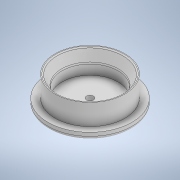
# Autodesk Inventor part: tale
Saved by Autodesk Inventor 2022 (Build 260153000, 153)
## iProperties
Created: 2023-01-18
Part Number: tale
Material: Generic
Document SubType Name: Modeling
Designer: CLCK
Density: 1 g/cm^3
Appearance: Default
Author: CLCK
Autodesk Inventor part; units mm, degrees
ref_plane "YZ Plane" through (0, 0, 0) normal (1, 0, 0) x (0, 1, 0)
ref_plane "XZ Plane" through (0, 0, 0) normal (0, 1, 0) x (-1, 0, 0)
ref_plane "XY Plane" through (0, 0, 0) normal (0, 0, 1) x (1, 0, 0)
sketch "Sketch1" plane through (0, 0, 0) normal (0, 1, 0) x (-1, 0, 0)
  circle A0 centre (0, 0) radius 6
  dimension "d0" = 12
  constraints: 1 centre point, 1 coincident
  measures "d0" diameter of A0
extrude "Extrusion1" add sketch "Sketch1" along normal blind 1
fillet "Fillet1" radius 0.5 1 edges at (6, 0, 0)
sketch "Sketch2" plane through (0, 1, 0) normal (0, 1, 0) x (1, 0, 0)
  circle A0 centre (0, 0) radius 0.5
  dimension "d4" = 1
  constraints: 1 centre point, 1 coincident
  measures "d4" diameter of A0
extrude "Extrusion2" cut sketch "Sketch2" against normal blind 1
sketch "Sketch3" plane through (0, 1, 0) normal (0, 1, 0) x (1, 0, 0)
  circle A0 centre (0, 0) radius 0.5 projected
  circle A1 centre (0, 0) radius 5
  circle A2 centre (0, 0) radius 4
  dimension "d7" = 10
  dimension "d8" = 8
  constraints: 2 centre point, 2 coincident
  measures "d7" diameter of A1
  measures "d8" diameter of A2
extrude "Extrusion3" add sketch "Sketch3" along normal blind 3 contours A1
chamfer "Chamfer1" distance 0.75 distance2 1.5 1 edges at (-4, 4, 0) measured on face at (4.5795, 4, 0.7179)
fillet "Fillet2" radius 0.2 1 edges at (-4.75, 4, 0)
fillet "Fillet3" radius 0.5 1 edges at (-4, 2.5, 0)
body "Solid1"
